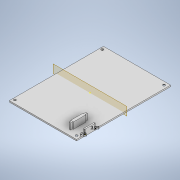
# Autodesk Inventor part: lower casing
Saved by Autodesk Inventor 2020.1 (Build 241239000, 239)
## iProperties
Created: 2019-06-23
Part Number: lower casing
Material: Generic
Document SubType Name: Modeling
Designer: jjsch
Density: 1 g/cm^3
Appearance: Default
Mass: 57.7992 g
Surface Area: 519.548 cm^2
Volume: 57.7992 cm^3
Author: jjsch
Autodesk Inventor part; units mm, degrees
ref_plane "YZ Plane" through (0, 0, 0) normal (1, 0, 0) x (0, 1, 0)
ref_plane "XZ Plane" through (0, 0, 0) normal (0, 1, 0) x (-1, 0, 0)
ref_plane "XY Plane" through (0, 0, 0) normal (0, 0, 1) x (1, 0, 0)
sketch "Sketch1" plane through (0, 0, 0) normal (0, 1, 0) x (-1, 0, 0)
  line L0 (-60, -84) -> (60, -84)
  line L1 (60, -84) -> (60, 84)
  line L2 (60, 84) -> (-60, 84)
  line L3 (-60, 84) -> (-60, -84)
  line L4 (-60, -84) -> (60, 84) construction
  line L5 (60, -84) -> (-60, 84) construction
  point P0 (0, 0)
  dimension "d0" = 168
  dimension "d1" = 120
  constraints: 12 end point, 2 midpoint, 2 parallel, 1 horizontal, 1 perpendicular
  measures "d0" distance of L1.end L0.end
  measures "d1" distance of L1.end L2.end
extrude "Extrusion1" add sketch "Sketch1" along normal blind 2.4
sketch "Sketch2" plane through (0, 2.4, 0) normal (0, 1, 0) x (1, 0, 0)
  line L0 (60, -84) -> (60, 84) projected
  line L1 (60, -68.75) -> (57.6, -68.75)
  line L2 (57.6, -68.75) -> (57.6, -51.25)
  line L3 (57.6, -51.25) -> (60, -51.25)
  line L4 (60, -51.25) -> (60, -68.75)
  line L5 (-60, -84) -> (60, -84) projected
  point P0 (0, 0)
  dimension "d4" = 2.4
  dimension "d5" = 17.5
  dimension "d6" = 15.25
  constraints: 8 end point, 2 parallel, 1 horizontal, 1 perpendicular, 1 point on line
  measures "d4" distance of L2.end L3.end
  measures "d5" distance of L1.end L2.end
  measures "d6" distance between parallel lines of L5 L1
extrude "Extrusion2" add sketch "Sketch2" along normal blind 8.25
sketch "Sketch3" plane through (0, 2.4, 0) normal (0, 1, 0) x (1, 0, 0)
  line L0 (59.425, -52.5) -> (58.175, -52.5)
  line L1 (58.175, -52.5) -> (58.175, -50)
  line L2 (58.175, -50) -> (59.425, -50)
  line L3 (59.425, -50) -> (59.425, -52.5)
  line L4 (57.6, -51.25) -> (60, -51.25) projected
  line L5 (59.425, -52.5) -> (58.175, -50) construction
  line L6 (58.175, -52.5) -> (59.425, -50) construction
  line L7 (59.425, -67.5) -> (58.175, -67.5)
  line L8 (58.175, -67.5) -> (58.175, -70)
  line L9 (58.175, -70) -> (59.425, -70)
  line L10 (59.425, -70) -> (59.425, -67.5)
  line L11 (60, -68.75) -> (57.6, -68.75) projected
  line L12 (59.425, -67.5) -> (58.175, -70) construction
  line L13 (58.175, -67.5) -> (59.425, -70) construction
  point P0 (0, 0)
  point P1 (58.8, -51.25)
  point P2 (58.8, -68.75)
  point P3 (59.425, -68.75)
  point P4 (58.175, -68.75)
  point P5 (58.175, -51.25)
  point P6 (59.425, -51.25)
  dimension "d9" = 1.25
  dimension "d10" = 2.5
  dimension "d11" = 1.25
  dimension "d12" = 2.5
  constraints: 24 end point, 6 midpoint, 4 parallel, 2 horizontal, 2 perpendicular
  measures "d9" distance of L1.end L2.end
  measures "d10" distance of L0.end L1.end
  measures "d11" distance of L9.end L8.end
  measures "d12" distance of L8.end L7.end
extrude "Extrusion3" add sketch "Sketch3" along normal blind 8.25 contours L4 L1 L2 L3 | L10 L9 L8 L11
sketch "Sketch4" plane through (0, 2.4, 0) normal (0, 1, 0) x (1, 0, 0)
  line L0 (60, -84) -> (60, -68.75) projected
  line L1 (-60, -84) -> (60, -84) projected
  line L2 (41.5, -71) -> (36.5, -71)
  line L3 (36.5, -71) -> (36.5, -49)
  line L4 (36.5, -49) -> (41.5, -49)
  line L5 (41.5, -49) -> (41.5, -71)
  line L6 (40.3125, -67) -> (37.6875, -67)
  line L7 (37.6875, -67) -> (37.6875, -75)
  line L8 (37.6875, -75) -> (40.3125, -75)
  line L9 (40.3125, -75) -> (40.3125, -67)
  line L10 (40.3125, -67) -> (37.6875, -75) construction
  line L11 (37.6875, -67) -> (40.3125, -75) construction
  line L12 (40.3125, -53) -> (37.6875, -53)
  line L13 (37.6875, -53) -> (37.6875, -45)
  line L14 (37.6875, -45) -> (40.3125, -45)
  line L15 (40.3125, -45) -> (40.3125, -53)
  line L16 (40.3125, -53) -> (37.6875, -45) construction
  line L17 (37.6875, -53) -> (40.3125, -45) construction
  point P0 (0, 0)
  point P1 (39, -71)
  point P2 (39, -49)
  point P3 (40.3125, -71)
  point P4 (37.6875, -71)
  point P5 (37.6875, -49)
  point P6 (40.3125, -49)
  dimension "d15" = 18.5
  dimension "d16" = 13
  dimension "d17" = 5
  dimension "d18" = 22
  dimension "d21" = 2.625
  dimension "d22" = 8
  dimension "d23" = 2.625
  dimension "d24" = 8
  constraints: 32 end point, 6 midpoint, 6 parallel, 3 horizontal, 3 perpendicular
  measures "d15" distance from line of L0 L2.start
  measures "d16" distance from line of L1 L2.start
  measures "d17" distance of L3.end L4.end
  measures "d18" distance of L2.end L3.end
  measures "d21" distance of L8.end L7.end
  measures "d22" distance of L7.end L6.end
  measures "d23" distance of L13.end L14.end
  measures "d24" distance of L12.end L13.end
extrude "Extrusion4" add sketch "Sketch4" along normal blind 11.25
ref_plane "Work Plane3" through (-60, 0, 0) normal (0, 0, 1) x (1, 0, 0)
sketch "Sketch11" plane through (0, 0, 0) normal (0, -1, 0) x (1, 0, 0)
  line L0 (-60, 84) -> (60, 84) projected
  line L1 (-60, -84) -> (-60, 84) projected
  line L2 (60, -84) -> (-60, -84) projected
  point P0 (0, 0)
  point P1 (-56, 78)
  point P2 (-56, -78)
  dimension "d63" = 6
  dimension "d64" = 4
  dimension "d65" = 4
  dimension "d66" = 6
  constraints: 1 vertical alignment
  measures "d63" distance from line of L0 point (-56, 78)
  measures "d64" distance from line of L1 point (-56, 78)
  measures "d65" distance from line of L1 point (-56, -78)
  measures "d66" distance from line of L2 point (-56, -78)
hole "Hole1" at (-56, 0, 78) at (-56, 0, -78) direction (0, 1, 0) diameter 4 end through all
sketch "Sketch12" plane through (0, 2.4, 0) normal (0, 1, 0) x (1, 0, 0)
  point P0 (0, 0)
sketch "Sketch13" plane through (0, 0, 0) normal (0, -1, 0) x (1, 0, 0)
  line L0 (60, 84) -> (60, -84) projected
  line L1 (-60, 84) -> (60, 84) projected
  point P0 (0, 0)
  point P1 (54, 78)
  point P2 (54.2858, -79.2517)
  dimension "d74" = 6
  dimension "d75" = 6
  measures "d74" distance from line of L0 point (54, 78)
  measures "d75" distance from line of L1 point (54, 78)
hole "Hole2" at (54, 0, 78) direction (0, 1, 0) diameter 4 depth 10 tip angle 118 countersink diameter 8.4 countersink angle 90
mirror "Mirror4" about plane through (-60, 0, 0) normal (0, 0, 1) of "Hole2"
body "Solid1"
